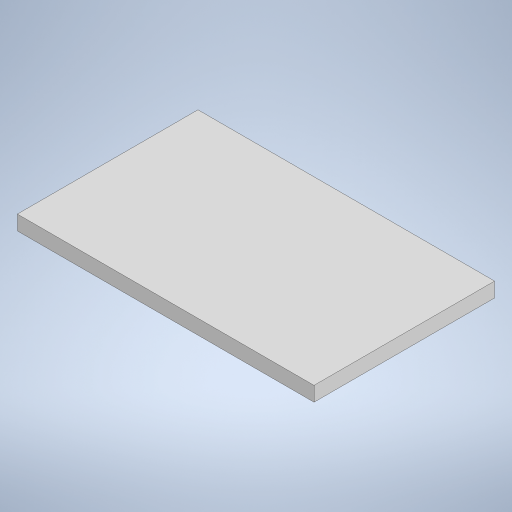
# Autodesk Inventor part: Base
Saved by Autodesk Inventor 2024 (Build 280153000, 153)
## iProperties
Created: 2023-10-07
Part Number: Base
Material: Generic
Document SubType Name: Modeling
Designer: chris
Density: 1 g/cm^3
Appearance: Default
Author: chris
Autodesk Inventor part; units mm, degrees
ref_plane "YZ Plane" through (0, 0, 0) normal (1, 0, 0) x (0, 1, 0)
ref_plane "XZ Plane" through (0, 0, 0) normal (0, 1, 0) x (-1, 0, 0)
ref_plane "XY Plane" through (0, 0, 0) normal (0, 0, 1) x (1, 0, 0)
sketch "Sketch1" plane through (0, 0, 0) normal (0, 1, 0) x (-1, 0, 0)
  line L0 (19.7838, 19.7838) -> (-19.7838, 19.7838)
  line L1 (-19.7838, 19.7838) -> (-19.7838, -19.7838)
  line L2 (-19.7838, -19.7838) -> (19.7838, -19.7838)
  line L3 (19.7838, -19.7838) -> (19.7838, 19.7838)
  line L4 (19.7838, 19.7838) -> (-19.7838, -19.7838) construction
  line L5 (-19.7838, 19.7838) -> (19.7838, -19.7838) construction
  line L6 (-19.7838, -19.7838) -> (-45.2162, -19.7838)
  line L7 (-45.2162, -19.7838) -> (-45.2162, 19.7838)
  line L8 (-45.2162, 19.7838) -> (-19.7838, 19.7838)
  line L9 (-19.7838, 19.7838) -> (-19.7838, -19.7838)
  point P0 (0, 0)
  dimension "d4" = 65
  constraints: 20 end point, 4 parallel, 3 perpendicular, 2 horizontal, 2 midpoint, 1 collinear
  measures "d4" distance between parallel lines of L3 L7
extrude "Extrusion1" add sketch "Sketch1" along normal blind 3.2
body "Solid1"
